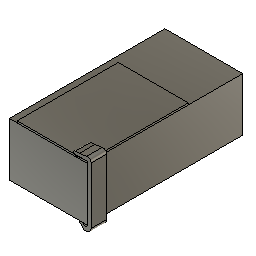
mouse-mat-to-ikea-table-clip (Autodesk Fusion 360 design; units mm, degrees)
Autodesk Fusion 360 part; units mm, degrees
sketch "Sketch1" plane through (0, 0, 0) normal (0, 1, 0) x (1, 0, 0) in component "table"
  line L0 (0, 0) -> (-50, 0)
  line L1 (-50, 0) -> (-50, 34.3)
  line L2 (-50, 34.3) -> (0, 34.3)
  line L3 (0, 34.3) -> (0, 0)
  dimension "d1" = 50
  dimension "d2" = 34.3
  constraint horizontal L0
  constraint vertical L1
  constraint horizontal L2
  constraint vertical L3
  constraint coincident L0.start L3.end
  measures "d1" distance of L0.start L0.end
  measures "d2" distance of L0.start L2.end
extrude "Extrude1" add sketch "Sketch1" along normal blind 100 makes body 1 in component "table"
sketch "Sketch1 (2)" plane through (0, 0, 0) normal (0, 0, 1) x (-1, 0, 0) in component "mouse-mat"
  line L0 (50, 0) -> (0, 0)
  line L1 (0, 0) -> (0, -100)
  line L2 (0, -100) -> (50, -100)
  line L3 (50, -100) -> (50, 0)
  line L4 (0, 0) -> (45, 0)
  line L5 (45, 0) -> (45, -65)
  line L6 (45, -65) -> (0, -65)
  line L7 (0, -65) -> (0, 0)
  constraint horizontal L4
  constraint vertical L5
  constraint horizontal L6
  constraint vertical L7
  constraint coincident L0.end L1.start
extrude "Extrude1'" add sketch "Sketch1 (2)" along normal blind 1.2 separate body contours L0 L1 L4 L5 L6 L7 makes body 2 in component "mouse-mat"
sketch "Sketch1 (3)" plane through (0, 0, 0) normal (0, -1, 0) x (1, 0, 0) in component "clip"
  line L0 (0, -34.3) -> (0, 0)
  line L1 (0, 0) -> (-50, 0)
  line L2 (-50, 0) -> (-50, -34.3)
  line L3 (-7.6004, 1) -> (-5.5332, 1)
  line L4 (-5.5332, 1) -> (-0.3386, 1.3346)
  line L5 (0, 1.0347) -> (0, -34.3)
  line L6 (-7.6004, 3) -> (-5.0582, 3)
  line L7 (-5.0582, 3) -> (-0.3212, 3.8008)
  arc A0 (2.5, 1.4165) -> (-0.3212, 3.8008) centre (0.0819, 1.4165) ccw
  line L8 (2.5, 1.4165) -> (2.5, -35)
  arc A1 (-7.6004, 3) -> (-7.6004, 1) centre (-7.6004, 2) ccw
  arc A2 (0, 1.0347) -> (-0.3386, 1.3346) centre (-0.3181, 1.0167) ccw
  arc A3 (-2.5, -35) -> (0, -34.3) centre (-1.348, -34.3) ccw
  arc A4 (-2.5, -35) -> (-5, -35) centre (-3.75, -35.7595) ccw
  arc A5 (-3.75, -35.7595) -> (2.5, -35) centre (-0.6712, -35) ccw
  arc A6 (-5, -35) -> (-4.4935, -35.7595) centre (-4.5695, -35.2616) ccw
  arc A7 (-3.75, -35.7595) -> (-4.4935, -35.7595) centre (-4.1218, -38.1964) ccw
  line L9 (-6, 1) -> (-6.8, 0.2)
  line L10 (-6.8, 0.2) -> (-7.6004, 1)
  dimension "d7" = 2
  constraint horizontal L3
  constraint parallel L0 L5
  constraint tangent L7 A0
  constraint tangent A0 L8
  constraint horizontal L6
  constraint tangent L6 A1
  constraint tangent L4 A2
  constraint coincident L0.start L5.end
  constraint tangent L5 A3
  constraint tangent A3 A4
  constraint coincident A4.centre A5.start
  constraint tangent L8 A5
  constraint tangent A4 A6
  constraint tangent A6 A7
  constraint coincident L3 L9.start
  measures "d7" distance of L3.start L6.start
extrude "Extrude1''" add sketch "Sketch1 (3)" against normal blind 10 separate body makes body 3 in component "clip"
component "table" placed x (1, 0, 0) y (0, 1, 0) z (0, 0, 1) at (0, 0, 0)
component "mouse-mat" placed x (1, 0, 0) y (0, 1, 0) z (0, 0, 1) at (0, 0, 0)
component "clip" placed x (1, 0, 0) y (0, 1, 0) z (0, 0, 1) at (0, 0, 0)
